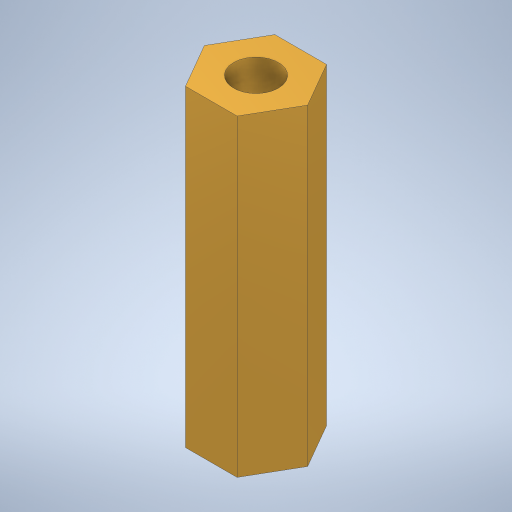
# Autodesk Inventor part: hex_spacer_14
Saved by Autodesk Inventor 2024.1 (Build 281209000, 209)
## iProperties
Created: 2023-11-11
Part Number: hex_spacer_14
Material: Générique
Document SubType Name: Modeling
Designer: Thibault
Density: 1 g/cm^3
Appearance: Par défaut
Author: Thibault
Autodesk Inventor part; units mm, degrees
ref_plane "YZ Plane" through (0, 0, 0) normal (1, 0, 0) x (0, 1, 0)
ref_plane "XZ Plane" through (0, 0, 0) normal (0, 1, 0) x (-1, 0, 0)
ref_plane "XY Plane" through (0, 0, 0) normal (0, 0, 1) x (1, 0, 0)
sketch "Esquisse1" plane through (0, 0, 0) normal (0, 1, 0) x (-1, 0, 0)
  line L0 (1.1547, -2) -> (-1.1547, -2)
  line L1 (-1.1547, -2) -> (-2.3094, 0)
  line L2 (-2.3094, 0) -> (-1.1547, 2)
  line L3 (-1.1547, 2) -> (1.1547, 2)
  line L4 (1.1547, 2) -> (2.3094, 0)
  line L5 (2.3094, 0) -> (1.1547, -2)
  circle A0 centre (0, 0) radius 1
  dimension "d0" = 2
  dimension "d1" = 2
  constraints: 12 end point, 2 coincident, 1 centre point, 1 horizontal, 13 other
  measures "d0" diameter of A0
  measures "d1" distance from line of point (0, 0) L4
extrude "Extrusion1" add sketch "Esquisse1" along normal blind 14
